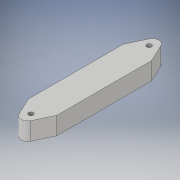
# Autodesk Inventor part: Rahmen_Y_Halterung_v1
Saved by Autodesk Inventor 2019 (Build 230136000, 136)
## iProperties
Created: 2018-08-18
Part Number: Rahmen_Y_Halterung_v1
Material: Generic
Document SubType Name: Modeling
Designer: Julia
Density: 1 g/cm^3
Appearance: Default
Author: Julia
Autodesk Inventor part; units mm, degrees
ref_plane "YZ Plane" through (0, 0, 0) normal (1, 0, 0) x (0, 1, 0)
ref_plane "XZ Plane" through (0, 0, 0) normal (0, 1, 0) x (-1, 0, 0)
ref_plane "XY Plane" through (0, 0, 0) normal (0, 0, 1) x (1, 0, 0)
sketch "Sketch1" plane through (0, 0, 0) normal (0, 1, 0) x (-1, 0, 0)
  circle A0 centre (0, 35) radius 7.5
  circle A1 centre (0, -35) radius 7.5
  circle A2 centre (0, 0) radius 6
  dimension "d0" = 15
  dimension "d1" = 35
  dimension "d2" = 15
  dimension "d3" = 35
  dimension "d4" = 12
  constraints: 3 centre point, 2 vertical alignment, 1 coincident
  measures "d0" diameter of A0
  measures "d1" distance of point (0, 0) A0.centre
  measures "d2" diameter of A1
  measures "d3" distance of point (0, 0) A1.centre
  measures "d4" diameter of A2
sketch "Sketch2" plane through (0, 0, 0) normal (0, 1, 0) x (-1, 0, 0)
  line L0 (12, 40) -> (12, -40)
  line L1 (12, -40) -> (5, -55)
  line L2 (12, 40) -> (5, 55)
  line L3 (0, 53.0774) -> (0, -54.9051) construction
  line L4 (-12, 40) -> (-12, -40)
  line L5 (-12, -40) -> (-5, -55)
  line L6 (-12, 40) -> (-5, 55)
  arc A0 (5, 55) -> (-5, 55) centre (0, 52.6667) ccw
  arc A1 (-5, -55) -> (5, -55) centre (0, -52.6667) ccw
  point P0 (0, 0)
  dimension "d5" = 12
  dimension "d6" = 40
  dimension "d7" = 40
  dimension "d8" = 15
  dimension "d9" = 7
  dimension "d10" = 15
  dimension "d11" = 7
  constraints: 14 end point, 4 point on circle, 4 symmetric about line, 4 tangent, 3 vertical, 2 centre point
  measures "d5" distance from line of L0 point (0, 0)
  measures "d6" vertical distance of point (0, 0) L0.end
  measures "d7" vertical distance of point (0, 0) L0.start
  measures "d8" vertical distance of L1.end L0.end
  measures "d9" horizontal distance of L1.end L0.end
  measures "d10" vertical distance of L2.end L0.start
  measures "d11" horizontal distance of L2.end L0.start
extrude "Extrusion1" add sketch "Sketch2" along normal blind 15
extrude "Extrusion2" cut sketch "Sketch1" along normal blind 10
sketch "Sketch3" plane through (0, 0, 0) normal (0, -1, 0) x (1, 0, 0)
  point P0 (0, 0)
  point P1 (0, -50)
  point P2 (0, 50)
  dimension "d16" = 50
  dimension "d17" = 50
  constraints: 2 vertical alignment
  measures "d16" distance of point (0, 0) point (0, -50)
  measures "d17" distance of point (0, 0) point (0, 50)
hole "Hole1" at (0, 0, -50) at (0, 0, 50) direction (0, 1, 0) diameter 4 end through all counterbore diameter 5 counterbore depth 2
body "Solid1"
